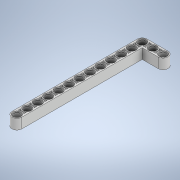
# Autodesk Inventor part: gear-rack
Saved by Autodesk Inventor 2021 (Build 250183000, 183)
## iProperties
Created: 2024-04-10
Part Number: gear-rack
Material: Generic
Document SubType Name: Modeling
Designer: 22hamfri
Density: 1 g/cm^3
Appearance: Default
Author: 22hamfri
Autodesk Inventor part; units mm, degrees
ref_plane "YZ Plane" through (0, 0, 0) normal (1, 0, 0) x (0, 1, 0)
ref_plane "XZ Plane" through (0, 0, 0) normal (0, 1, 0) x (-1, 0, 0)
ref_plane "XY Plane" through (0, 0, 0) normal (0, 0, 1) x (1, 0, 0)
sketch "Sketch1" plane through (0, 0, 0) normal (0, 1, 0) x (-1, 0, 0)
  circle A0 centre (0, 0) radius 2.575
  circle A1 centre (0, 0) radius 3.1
  circle A2 centre (0, 0) radius 3.8
  line L0 (0, 0) -> (-15.94, 0)
  circle A3 centre (-7.97, 0) radius 2.575
  circle A4 centre (-7.97, 0) radius 3.1
  circle A5 centre (-7.97, 0) radius 3.8
  circle A6 centre (-15.94, 0) radius 2.575
  circle A7 centre (-15.94, 0) radius 3.1
  circle A8 centre (-15.94, 0) radius 3.8
  line L1 (0, 0) -> (0, 95.64)
  circle A9 centre (0, 7.97) radius 2.575
  circle A10 centre (0, 7.97) radius 3.1
  circle A11 centre (0, 7.97) radius 3.8
  circle A12 centre (0, 15.94) radius 2.575
  circle A13 centre (0, 15.94) radius 3.1
  circle A14 centre (0, 15.94) radius 3.8
  circle A15 centre (0, 23.91) radius 2.575
  circle A16 centre (0, 23.91) radius 3.1
  circle A17 centre (0, 23.91) radius 3.8
  circle A18 centre (0, 31.88) radius 2.575
  circle A19 centre (0, 31.88) radius 3.1
  circle A20 centre (0, 31.88) radius 3.8
  circle A21 centre (0, 39.85) radius 2.575
  circle A22 centre (0, 39.85) radius 3.1
  circle A23 centre (0, 39.85) radius 3.8
  circle A24 centre (0, 47.82) radius 2.575
  circle A25 centre (0, 47.82) radius 3.1
  circle A26 centre (0, 47.82) radius 3.8
  circle A27 centre (0, 55.79) radius 2.575
  circle A28 centre (0, 55.79) radius 3.1
  circle A29 centre (0, 55.79) radius 3.8
  circle A30 centre (0, 63.76) radius 2.575
  circle A31 centre (0, 63.76) radius 3.1
  circle A32 centre (0, 63.76) radius 3.8
  circle A33 centre (0, 71.73) radius 2.575
  circle A34 centre (0, 71.73) radius 3.1
  circle A35 centre (0, 71.73) radius 3.8
  circle A36 centre (0, 79.7) radius 2.575
  circle A37 centre (0, 79.7) radius 3.1
  circle A38 centre (0, 79.7) radius 3.8
  circle A39 centre (0, 87.67) radius 2.575
  circle A40 centre (0, 87.67) radius 3.1
  circle A41 centre (0, 87.67) radius 3.8
  circle A42 centre (0, 95.64) radius 2.575
  circle A43 centre (0, 95.64) radius 3.1
  circle A44 centre (0, 95.64) radius 3.8
  line L2 (-3.8, 95.64) -> (-3.8, 3.8)
  line L3 (-3.8, 3.8) -> (-15.94, 3.8)
  line L4 (-15.94, -3.8) -> (0, -3.8)
  line L5 (3.8, 0) -> (3.8, 95.64)
  line L6 (2.3, 92.6151) -> (2.3, 90.6949)
  line L7 (2.3, 84.6451) -> (2.3, 82.7249)
  line L8 (2.3, 76.6751) -> (2.3, 74.7549)
  line L9 (2.3, 68.7051) -> (2.3, 66.7849)
  line L10 (2.3, 60.7351) -> (2.3, 58.8149)
  line L11 (2.3, 52.7651) -> (2.3, 50.8449)
  line L12 (2.3, 44.7951) -> (2.3, 42.8749)
  line L13 (2.3, 36.8251) -> (2.3, 34.9049)
  line L14 (2.3, 28.8551) -> (2.3, 26.9349)
  line L15 (2.3, 20.8851) -> (2.3, 18.9649)
  line L16 (2.3, 12.9151) -> (2.3, 10.9949)
  line L17 (2.3, 4.9451) -> (2.3, 3.0249)
  line L18 (-3.0249, -2.3) -> (-4.9451, -2.3)
  line L19 (-10.9949, -2.3) -> (-12.9151, -2.3)
  line L20 (-12.9151, 2.3) -> (-10.9949, 2.3)
  line L21 (-4.9451, 2.3) -> (-3.0249, 2.3)
  line L22 (-2.3, 3.0249) -> (-2.3, 4.9451)
  line L23 (-2.3, 10.9949) -> (-2.3, 12.9151)
  line L24 (-2.3, 18.9649) -> (-2.3, 20.8851)
  line L25 (-2.3, 26.9349) -> (-2.3, 28.8551)
  line L26 (-2.3, 34.9049) -> (-2.3, 36.8251)
  line L27 (-2.3, 42.8749) -> (-2.3, 44.7951)
  line L28 (-2.3, 50.8449) -> (-2.3, 52.7651)
  line L29 (-2.3, 58.8149) -> (-2.3, 60.7351)
  line L30 (-2.3, 66.7849) -> (-2.3, 68.7051)
  line L31 (-2.3, 74.7549) -> (-2.3, 76.6751)
  line L32 (-2.3, 82.7249) -> (-2.3, 84.6451)
  line L33 (-2.3, 90.6949) -> (-2.3, 92.6151)
  dimension "d0" = 0.7
  dimension "d1" = 6.2
  dimension "d2" = 5.15
  dimension "d5" = 7.97
  dimension "d12" = 7.97
  dimension "d17" = 1.5
  dimension "d18" = 1.5
  dimension "d19" = 1.5
  dimension "d20" = 1.5
  constraints: 68 end point, 62 point on circle, 48 point on line, 45 centre point, 7 tangent, 5 vertical, 4 horizontal, 3 coincident, 56 other
  measures "d0" radial gap between concentric circles of A1 A2
  measures "d1" diameter of A1
  measures "d2" diameter of A0
  measures "d5" distance of L0.start A3.centre
  measures "d12" distance of L0.start A9.centre
  measures "d17" distance between parallel lines of L33 L2
  measures "d18" distance between parallel lines of L5 L6
  measures "d19" distance between parallel lines of L4 L19
  measures "d20" distance between parallel lines of L20 L3
extrude "Extrusion1" add sketch "Sketch1" against normal mid plane 7.76 contours L1 A2 L0 A1 | A1 L0 A2 L1 | L17 A11 L5 A2 | A2 L21 A5 L3 L2 A11 L22 | A11 L1 A10 | L1 A10 A11 | A2 L4 A5 L18 | A5 L0 A4 | L0 A4 A5 | A11 L16 A14 L5 | L2 A14 L23 A11 | A5 L20 A8 L3 | L4 A8 L19 A5 | A14 L1 A13 | A14 L15 A17 L5 | L2 A17 L24 A14 | A14 L1 A13 | A8 | A17 L1 A16 | A17 L14 A20 L5 | L2 A20 L25 A17 | A17 L1 A16 | A20 L1 A19 | A20 L13 A23 L5 | L2 A23 L26 A20 | A20 L1 A19 | A23 L1 A22 | A23 L12 A26 L5 | L2 A26 L27 A23 | A23 L1 A22 | A26 L1 A25 | A26 L11 A29 L5 | L2 A29 L28 A26 | A26 L1 A25 | A29 L1 A28 | A29 L10 A32 L5 | L2 A32 L29 A29 | A29 L1 A28 | A32 L1 A31 | A32 L9 A35 L5 | L2 A35 L30 A32 | A32 L1 A31 | A35 L1 A34 | A35 L8 A38 L5 | L2 A38 L31 A35 | A35 L1 A34 | A38 L1 A37 | A38 L7 A41 L5 | L2 A41 L32 A38 | A38 L1 A37 | A41 L1 A40 | A41 L6 A44 L5 | L2 A44 L33 A41 | A41 L1 A40 | A44
extrude "Extrusion2" add sketch "Sketch1" along normal mid plane 6.16 contours A0 L1 A1 L0 | A0 L0 A1 L1 | A10 L1 A9 | L1 A9 A10 | A4 L0 A3 | L0 A3 A4 | A13 L1 A12 | L1 A12 A13 | A16 L1 A15 | L1 A15 A16 | A19 L1 A18 | L1 A18 A19 | A22 L1 A21 | L1 A21 A22 | A25 L1 A24 | L1 A24 A25 | A28 L1 A27 | L1 A27 A28 | A31 L1 A30 | L1 A30 A31 | A34 L1 A33 | L1 A33 A34 | A37 L1 A36 | L1 A36 A37 | A40 L1 A39 | L1 A39 A40 | A7 | A43
extrude "Extrusion3" add sketch "Sketch1" along normal mid plane 4 contours L1 A11 L17 A2 | A2 L22 A11 L1 | L0 A5 L21 A2 | A2 L18 A5 L0 | A11 L1 A14 L16 | L23 A14 L1 A11 | A5 L0 A8 L20 | L19 A8 L0 A5 | A14 L1 A17 L15 | L24 A17 L1 A14 | A17 L1 A20 L14 | L25 A20 L1 A17 | A20 L1 A23 L13 | L26 A23 L1 A20 | A23 L1 A26 L12 | L27 A26 L1 A23 | A26 L1 A29 L11 | L28 A29 L1 A26 | A29 L1 A32 L10 | L29 A32 L1 A29 | A32 L1 A35 L9 | L30 A35 L1 A32 | A35 L1 A38 L8 | L31 A38 L1 A35 | A38 L1 A41 L7 | L32 A41 L1 A38 | A41 L1 A44 L6 | L33 A44 L1 A41
body "Solid1"
